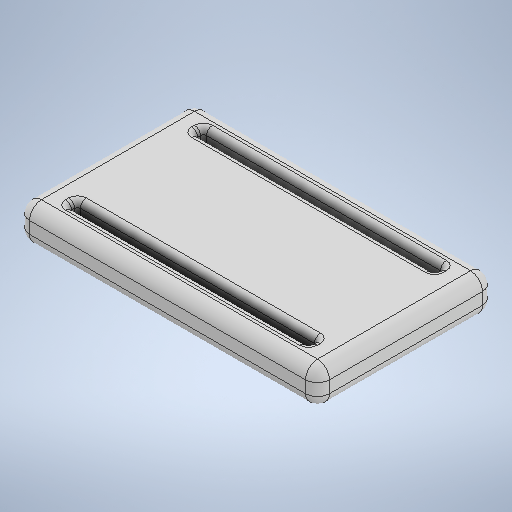
# Autodesk Inventor part: Trimming Template
Saved by Autodesk Inventor 2025.3 (Build 293356000, 356)
## iProperties
Created: 2025-05-10
Part Number: Trimming Template
Material: Generic
Document SubType Name: Modeling
Designer: vncnt
Density: 1 g/cm^3
Appearance: Default
Author: vncnt
## iProperties of the stored document Trimming Template_3DPrint.ipt
Created: 2025-05-10
Part Number: Trimming Template_3DPrint
Material: Generic
Document SubType Name: Modeling
Designer: vncnt
Density: 1 g/cm^3
Appearance: Default
Author: vncnt
Autodesk Inventor part; units mm, degrees
ref_plane "YZ Plane" through (0, 0, 0) normal (1, 0, 0) x (0, 1, 0)
ref_plane "XZ Plane" through (0, 0, 0) normal (0, 1, 0) x (-1, 0, 0)
ref_plane "XY Plane" through (0, 0, 0) normal (0, 0, 1) x (1, 0, 0)
sketch "Sketch1" plane through (0, 0, 0) normal (0, 1, 0) x (-1, 0, 0)
  line L0 (20, 9.75) -> (-20, 9.75)
  line L1 (-20, 9.75) -> (-20, -9.75)
  line L2 (-20, -9.75) -> (20, -9.75)
  line L3 (20, -9.75) -> (20, 9.75)
  line L4 (20, 9.75) -> (-20, -9.75) construction
  line L5 (-20, 9.75) -> (20, -9.75) construction
  line L6 (21.5, 11.25) -> (-21.5, 11.25)
  line L7 (-21.5, 11.25) -> (-21.5, -11.25)
  line L8 (-21.5, -11.25) -> (21.5, -11.25)
  line L9 (21.5, -11.25) -> (21.5, 11.25)
  line L10 (-20, 11.25) -> (20, 11.25)
  line L11 (20, 11.25) -> (20, -11.25)
  line L12 (20, -11.25) -> (-20, -11.25)
  line L13 (-20, -11.25) -> (-20, 11.25)
  line L14 (-20, 11.25) -> (20, -11.25) construction
  line L15 (20, 11.25) -> (-20, -11.25) construction
  line L16 (25, 14.75) -> (-25, 14.75)
  line L17 (-25, 14.75) -> (-25, -14.75)
  line L18 (-25, -14.75) -> (25, -14.75)
  line L19 (25, -14.75) -> (25, 14.75)
  point P0 (0, 0)
  point P1 (-19.6517, -9.75)
  dimension "d0" = 40
  dimension "d1" = 19.5
  dimension "d2" = 1.5
  dimension "d3" = 3.5
  constraints: 40 end point, 8 parallel, 4 midpoint, 4 perpendicular, 2 horizontal, 2 point on line, 6 other
  measures "d0" distance of L2.end L1.end
  measures "d1" distance of L1.end L0.end
  measures "d2" distance between parallel lines of L3 L9
  measures "d3" distance between parallel lines of L9 L19
extrude "Extrusion1" add sketch "Sketch1" along normal blind 6 contours L3 L2 L1 L0 | L11 L6 L9 L8 L3 | L1 L13 L8 L7 L6 | L19 L18 L17 L16
fillet "Fillet1" radius 2 12 edges at (0, 6, 14.75) (0, 0, 14.75) (25, 0, 0) (25, 6, 0) (0, 6, -14.75) (0, 0, -14.75) (-25, 0, 0) (-25, 6, 0) (-25, 3, 14.75) (-25, 3, -14.75) (25, 3, -14.75) (25, 3, 14.75)
fillet "Fillet2" radius 0.5 8 edges at (-20, 3, 9.75) (-20, 3, 11.25) (-20, 3, -9.75) (-20, 3, -11.25) (20, 3, -11.25) (20, 3, 9.75) (20, 3, 11.25) (20, 3, -9.75)
fillet "Fillet3" radius 1 30 edges at (-19.8536, 6, -9.8964) (-20, 6, -10.5) (-19.8536, 6, -11.1036) (0, 6, -11.25) (19.8536, 6, -11.1036) (20, 6, -10.5) (20, 6, 10.5) (0, 6, -9.75) (19.8536, 6, 9.8964) (19.8536, 6, 11.1036) (0, 6, 11.25) (-19.8536, 6, 11.1036) (-20, 6, 10.5) (-19.8536, 6, 9.8964) (0, 6, 9.75) (19.8536, 0, 9.8964) (20, 0, 10.5) (19.8536, 0, 11.1036) (0, 0, 11.25) (-19.8536, 0, 11.1036) (-20, 0, 10.5) (-19.8536, 0, 9.8964) (0, 0, 9.75) (-19.8536, 0, -9.8964) (-20, 0, -10.5) (-19.8536, 0, -11.1036) (0, 0, -11.25) (19.8536, 0, -11.1036) (20, 0, -10.5) (0, 0, -9.75)
body "Solid1"
